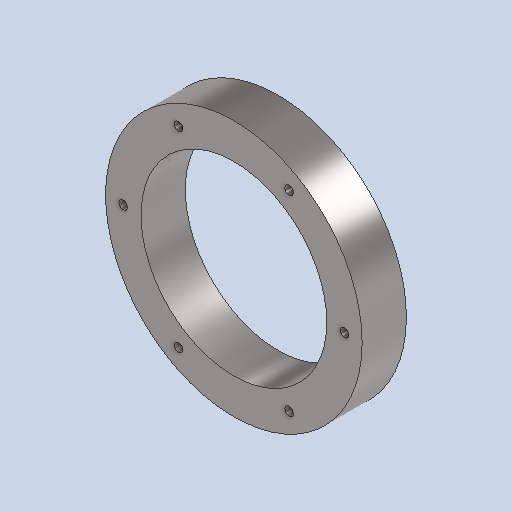
# Autodesk Inventor part: Część5
Saved by Autodesk Inventor 2024 (Build 280153000, 153)
## iProperties
Created: 2023-11-21
Part Number: Część5
Material: Stal nierdzewna
Document SubType Name: Modeling
Designer: Wojciech
Density: 8 g/cm^3
Appearance: Częściowo polerowany
Author: Wojciech
Autodesk Inventor part; units mm, degrees
ref_plane "YZ Plane" through (0, 0, 0) normal (1, 0, 0) x (0, 1, 0)
ref_plane "XZ Plane" through (0, 0, 0) normal (0, 1, 0) x (-1, 0, 0)
ref_plane "Płaszczyzna konstrukcyjna1" through (0, 0, 0) normal (0, 0, 1) x (1, 0, 0)
sketch "Szkic1" plane through (0, 0, 0) normal (0, 0, 1) x (1, 0, 0)
  circle A0 centre (0, 0) radius 72.5 projected
  circle A1 centre (0, 0) radius 52.5 projected
extrude "Wyciągnięcie proste1" add sketch "Szkic1" against normal blind 25
sketch "Szkic2" plane through (0, 0, -25) normal (0, 0, -1) x (-1, 0, 0)
  circle A0 centre (0, 0) radius 52.5 projected
  line L0 (-52.5, 0) -> (-72.5, 0)
  circle A1 centre (0, 0) radius 72.5 projected
  circle A2 centre (-62.5, 0) radius 3
  dimension "d2" = 20
  dimension "d3" = 6
  constraints: 2 end point, 2 horizontal alignment, 1 centre point, 1 horizontal, 1 midpoint, 2 other
  measures "d2" distance of L0.start L0.end
  measures "d3" diameter of A2
hole "Otwór1" at (62.5, 0, -25) direction (0, 0, 1) diameter 4.917 end through all thread size "M6x1" class "6H" standard "ISO Metric profile"
pattern_circular "Szyk kołowy1" count 6 over 360 about axis through (0, 0, -10) along (0, 0, 1) of "Otwór1"
